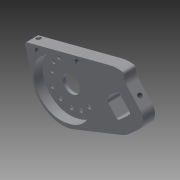
# Autodesk Inventor part: mount_alt_2015
Saved by Autodesk Inventor 2015 (Build 190159000, 159)
## iProperties
Created: 2014-05-15
Part Number: mount_alt_2015
Material: Generic
Document SubType Name: Modeling
Designer: brent
Density: 1 g/cm^3
Appearance: Default
Author: brent
Autodesk Inventor part; units mm, degrees
ref_plane "YZ Plane" through (0, 0, 0) normal (1, 0, 0) x (0, 1, 0)
ref_plane "XZ Plane" through (0, 0, 0) normal (0, 1, 0) x (-1, 0, 0)
ref_plane "XY Plane" through (0, 0, 0) normal (0, 0, 1) x (1, 0, 0)
derived "mountsketch_alt.ipt"
sketch "Sketch1" plane through (0, 0, 0) normal (0, 0, 1) x (1, 0, 0)
  circle A0 centre (-32.7716, 175.7429) radius 9 projected
  circle A1 centre (-51.4977, 187.2899) radius 2.15 projected
  circle A2 centre (-32.7716, 175.7429) radius 33 projected
  circle A3 centre (-44.3186, 157.0168) radius 2.15 projected
  circle A4 centre (-14.0455, 164.1958) radius 2.15 projected
  circle A5 centre (-21.2245, 194.4689) radius 2.15 projected
  line L0 (127, 127.3759) -> (61.9125, 127.3759) projected
  line L1 (-105.8581, 0) -> (165.8097, 0) projected
  line L2 (32.8717, 216.1784) -> (58.0256, 188.2421) projected
  line L3 (58.0256, 188.2421) -> (34.4308, 166.9972) projected
  line L4 (-21.2245, 194.4689) -> (-14.0455, 164.1958) projected
  line L5 (-32.7716, 175.7429) -> (26.1158, 189.7076) projected
  line L6 (26.1158, 189.7076) -> (-31.1651, 176.1238) projected
  circle A6 centre (-9.2209, 174.5577) radius 2.15 projected
  line L7 (26.1158, 189.7076) -> (-34.378, 175.3619) projected
  circle A7 centre (-22.6931, 156.7216) radius 2.15 projected
  circle A8 centre (-29.599, 198.068) radius 2.15 projected
  circle A9 centre (-53.1093, 177.6899) radius 2.15 projected
  circle A10 centre (-32.7312, 154.1796) radius 2.15 projected
  circle A11 centre (-15.7377, 187.0468) radius 2.15 projected
  circle A12 centre (-46.063, 194.0022) radius 2.15 projected
  circle A13 centre (-53.0184, 163.6769) radius 2.15 projected
  line L8 (16.1602, 187.2887) -> (24.9131, 177.5677) projected
  line L9 (25.6305, 177.5301) -> (38.2774, 188.9173) projected
  line L10 (38.315, 189.6348) -> (29.5621, 199.3558) projected
  line L11 (32.8717, 216.1784) -> (-36.3872, 208.5442) projected
  line L12 (34.4308, 166.9972) -> (-20.5563, 145.0869) projected
  circle A14 centre (26.1158, 189.7076) radius 34.33 projected
  line L13 (32.8717, 216.1784) -> (32.0626, 223.5186) projected
  line L14 (26.8329, 203.9052) -> (40.0897, 189.182) projected
  line L15 (16.1602, 187.2887) -> (25.9328, 176.4351) projected
  line L16 (25.9328, 176.4351) -> (40.0897, 189.182) projected
  line L17 (26.8329, 203.9052) -> (19.3412, 197.1596) projected
  ellipse E0 centre (22.8611, 193.3223) end of major axis (29.5621, 199.3558) minor radius 5.2071 (19.3412, 197.1596) -> (16.1602, 187.2887) ccw projected
  line L18 (-41.0899, 207.6772) -> (17.4623, 222.929) projected
  line L19 (-41.0899, 207.6772) -> (-73.0243, 199.3589) projected
  line L20 (-73.0243, 199.3589) -> (-64.706, 167.4245) projected
  point P0 (0, 0)
  point P1 (-2.1526, 151.7421)
  point P2 (-5.3493, 194.1009)
  point P3 (0.5466, 212.6153)
  constraints: 4 other
extrude "Extrusion11" add sketch "Sketch1" along normal blind 12.7 contours A2 A14 | L11 A14 A2 | A2 L18 A14 L11 | A2 L20 L19 | A14 L11 L2 L3 L12 A2 | A2 L5 A14 | A14 L13 L11 | A2 A14 L5 | A2 A14 L12
fillet "Fillet7" radius 25.4 1 edges at (34.4308, 166.9972, 6.35)
fillet "Fillet7" radius 2.54 1 edges at (32.0626, 223.5186, 6.35)
fillet "Fillet7" radius 12.7 2 edges at (58.0256, 188.2421, 6.35) (32.8717, 216.1784, 6.35)
sketch "Sketch17" plane through (-32.7716, 175.7429, 12.7) normal (0, 0, 1) x (0.4514581, 0.8922923, 0)
  circle A0 centre (9.5746, -21.5491) radius 2.15 projected
  circle A1 centre (0, 0) radius 9 projected
  circle A2 centre (-12.4225, -17.5803) radius 2.15 projected
  circle A3 centre (-19.9069, 12.6188) radius 2.15 projected
  circle A4 centre (10.2922, 20.1032) radius 2.15 projected
  circle A5 centre (17.7766, -10.0959) radius 2.15 projected
  circle A6 centre (-19.2225, -9.7709) radius 2.15 projected
  circle A7 centre (-7.4443, 19.0262) radius 2.15 projected
  circle A8 centre (21.3528, 7.248) radius 2.15 projected
  circle A9 centre (21.9221, -1.8493) radius 2.15 projected
  circle A10 centre (-1.8493, -21.9221) radius 2.15 projected
  circle A11 centre (-21.9221, 1.8493) radius 2.15 projected
  circle A12 centre (1.8493, 21.9221) radius 2.15 projected
  arc A13 (-22.1213, -18.6795) -> (22.1213, 18.6795) centre (1.0652, -1.2614) ccw
  arc A14 (22.1213, 18.6795) -> (-22.1213, -18.6795) centre (-1.0652, 1.2614) ccw
  line L0 (-21.0921, -19.9712) -> (-23.2224, -17.4484)
  line L1 (23.2224, 17.4484) -> (21.0921, 19.9712)
  point P0 (65.9055, 28.4481)
  point P1 (29.8536, 27.856)
  point P2 (5.2355, 34.1004)
  point P3 (-142.019, -108.5824)
  point P4 (3.0016, 34.3692)
  dimension "d178" = 58
  dimension "d179" = 58
  constraints: 8 point on circle, 4 end point, 4 tangent, 2 centre point, 2 coincident
  measures "d178" diameter of A14
  measures "d179" diameter of A13
sketch "Sketch12" plane through (49.5277, 197.68, 12.7) normal (0.7431448, 0.6691306, 0) x (0, 0, -1)
  line L0 (12.7, 0) -> (12.7, 20.801) projected
  line L1 (12.7, 13.589) -> (12.7, 0) projected
  line L2 (12.7, 13.589) -> (0, 13.589) projected
  line L3 (0, 0) -> (0, 13.589) projected
  line L4 (12.7, 0) -> (0, 0) projected
  circle A0 centre (6.35, 9.525) radius 2.413
  line L5 (12.7, 14.605) -> (12.7, 0) projected
  line L6 (12.7, 14.605) -> (0, 14.605) projected
  line L7 (0, 0) -> (0, 14.605) projected
  line L8 (12.7, 0) -> (0, 0) projected
  point P0 (12.7, -113.7644)
  dimension "d99" = 4.826
  dimension "d122" = 6.35
  dimension "d123" = 5.08
  constraints: 1 centre point
  measures "d99" diameter of A0
  measures "d122" distance from line of L0 A0.centre
  measures "d123" distance from line of L6 A0.centre
sketch "Sketch13" plane through (48.5877, 179.7441, 0) normal (0.6691306, -0.7431448, 0) x (0.7431448, 0.6691306, 0)
  line L0 (-14.5085, 12.7) -> (0, 12.7) projected
  line L1 (-18.034, 0) -> (0, 0) projected
  line L2 (-18.034, 0) -> (-18.034, 12.7) projected
  line L3 (0, 12.7) -> (-18.034, 12.7) projected
  line L4 (0, 0) -> (0, 12.7) projected
  circle A0 centre (-9.017, 6.35) radius 2.413
  point P0 (-156.38, 0)
  dimension "d100" = 4.826
  dimension "d101" = 9.017
  dimension "d102" = 6.35
  constraints: 1 centre point
  measures "d100" diameter of A0
  measures "d101" distance from line of A0.centre L4
  measures "d102" distance from line of A0.centre L0
extrude "Extrusion13" cut sketch "Sketch13" against normal blind 25.4 contours A0
extrude "Extrusion14" cut sketch "Sketch12" against normal blind 25.4 contours A0
thread "Thread5" size "10-32 UNF" class "2B" standard "ANSI Unified Screw Threads" full length
thread "Thread6" size "10-32 UNF" class "2B" standard "ANSI Unified Screw Threads" full length
sketch "Sketch16" plane through (-32.7716, 175.7429, 0) normal (0, 0, -1) x (-0.4514581, -0.8922923, 0)
  line L0 (-38.0971, 0.9443) -> (-44.0427, -11.275) projected
  line L1 (-44.0427, -11.275) -> (-60.259, -3.3847) projected
  line L2 (-60.259, -3.3847) -> (-54.3134, 8.8346) projected
  arc A0 (-64.2386, -44.1331) -> (-64.2386, -44.1331) centre (-76.0821, -48.718) ccw projected
  line L3 (-56.729, -63.5313) -> (-64.2386, -44.1331) projected
  arc A1 (-56.729, -63.5313) -> (-40.3006, -70.7899) centre (-44.8855, -58.9464) ccw projected
  line L4 (-26.7706, -65.552) -> (-40.3006, -70.7899) projected
  arc A2 (-26.7706, -65.552) -> (-19.1307, -60.9069) centre (-35.9404, -41.865) ccw projected
  line L5 (21.8394, -24.7394) -> (-19.1307, -60.9069) projected
  arc A3 (21.8394, -24.7394) -> (21.8394, 24.7394) centre (0, 0) ccw projected
  line L6 (-34.7521, 29.5687) -> (-5.2355, 34.1004) projected
  circle A4 centre (-1.8493, 21.9221) radius 2.15 projected
  circle A5 centre (21.9221, 1.8493) radius 2.15 projected
  circle A6 centre (1.8493, -21.9221) radius 2.15 projected
  circle A7 centre (-21.9221, -1.8493) radius 2.15 projected
  circle A8 centre (-21.3528, 7.248) radius 2.15 projected
  circle A9 centre (7.4443, 19.0262) radius 2.15 projected
  circle A10 centre (19.2225, -9.7709) radius 2.15 projected
  circle A11 centre (-17.7766, -10.0959) radius 2.15 projected
  circle A12 centre (-10.2922, 20.1032) radius 2.15 projected
  circle A13 centre (19.9069, 12.6188) radius 2.15 projected
  circle A14 centre (12.4225, -17.5803) radius 2.15 projected
  circle A15 centre (-9.5746, -21.5491) radius 2.15 projected
  circle A16 centre (0, 0) radius 9 projected
  line L7 (-70.2544, 22.6003) -> (-60.2386, -42.6353)
  line L8 (-60.2386, -42.6353) -> (37.6257, -27.6099)
  line L9 (37.6257, -27.6099) -> (27.6099, 37.6257)
  line L10 (27.6099, 37.6257) -> (-70.2544, 22.6003)
  point P0 (-51.5181, 22.1934)
  point P1 (-5.2355, 34.1004)
  point P2 (142.019, -108.5824)
  point P3 (-29.8536, 27.856)
  point P4 (-65.9055, 28.4481)
  point P5 (-30.9895, -27.5591)
  point P6 (-69.1415, -38.0823)
  point P7 (-3.0016, 34.3692)
  dimension "d117" = 99.011
  dimension "d118" = 66
  constraints: 8 end point, 2 parallel, 1 perpendicular, 1 tangent, 9 other
  measures "d117" distance between parallel lines of L9 L7
  measures "d118" distance between parallel lines of L10 L8
extrude "Extrusion15" cut sketch "Sketch17" against normal blind 9.525 contours A14 A13
fillet "Fillet8" radius 2.3813 3 edges at (26.8329, 203.9052, 6.35) (40.0897, 189.182, 6.35) (25.9328, 176.4351, 6.35)
fillet "Fillet9" radius 2.54 1 edges at (-73.0243, 199.3589, 6.35)
sketch "Sketch18" plane through (-32.7716, 175.7429, 0) normal (0, 0, -1) x (-0.4514581, -0.8922923, 0)
  arc A0 (-56.729, -63.5313) -> (-40.3006, -70.7899) centre (-44.8855, -58.9464) ccw projected
  line L0 (-26.7706, -65.552) -> (-40.3006, -70.7899) projected
  arc A1 (-26.7706, -65.552) -> (-19.1307, -60.9069) centre (-35.9404, -41.865) ccw projected
  line L1 (21.8394, -24.7394) -> (-19.1307, -60.9069) projected
  arc A2 (21.8394, -24.7394) -> (21.8394, 24.7394) centre (0, 0) ccw projected
  line L2 (-34.7521, 29.5687) -> (-5.2355, 34.1004) projected
  arc A3 (-41.8032, 30.5011) -> (-34.7521, 29.5687) centre (-36.6794, 42.1216) ccw projected
  arc A4 (-64.7823, -23.5207) -> (-71.2503, -34.3482) centre (-39.0458, -46.2403) ccw projected
  arc A5 (-71.2503, -34.3482) -> (-70.2556, -37.3552) centre (-68.8675, -35.2281) ccw projected
  line L3 (-69.1415, -38.0823) -> (-70.2556, -37.3552) projected
  arc A6 (-64.2386, -44.1331) -> (-64.2386, -44.1331) centre (-76.0821, -48.718) ccw projected
  line L4 (-56.729, -63.5313) -> (-64.2386, -44.1331) projected
  circle A7 centre (-1.8493, 21.9221) radius 2.15 projected
  circle A8 centre (21.9221, 1.8493) radius 2.15 projected
  circle A9 centre (1.8493, -21.9221) radius 2.15 projected
  circle A10 centre (-21.9221, -1.8493) radius 2.15 projected
  circle A11 centre (-21.3528, 7.248) radius 2.15 projected
  circle A12 centre (7.4443, 19.0262) radius 2.15 projected
  circle A13 centre (19.2225, -9.7709) radius 2.15 projected
  circle A14 centre (-17.7766, -10.0959) radius 2.15 projected
  circle A15 centre (-10.2922, 20.1032) radius 2.15 projected
  circle A16 centre (19.9069, 12.6188) radius 2.15 projected
  circle A17 centre (12.4225, -17.5803) radius 2.15 projected
  circle A18 centre (0, 0) radius 9 projected
  circle A19 centre (-9.5746, -21.5491) radius 2.15 projected
  ellipse E0 centre (-40.8018, -41.7042) end of major axis (-49.2107, -44.9595) minor radius 5.2071 (-32.3929, -38.4489) -> (-42.6367, -36.831) ccw projected
  line L5 (-32.3929, -38.4489) -> (-27.98, -49.8483) projected
  arc A20 (-29.3409, -52.9286) -> (-27.98, -49.8483) centre (-30.2006, -50.708) ccw projected
  line L6 (-29.3409, -52.9286) -> (-42.6649, -58.0867) projected
  arc A21 (-45.7452, -56.7257) -> (-42.6649, -58.0867) centre (-43.5245, -55.866) ccw projected
  line L7 (-45.7452, -56.7257) -> (-51.1783, -42.6912) projected
  arc A22 (-49.8174, -39.6108) -> (-51.1783, -42.6912) centre (-48.9577, -41.8315) ccw projected
  line L8 (-49.8174, -39.6108) -> (-42.6367, -36.831) projected
  line L9 (-85.8325, -31.7522) -> (-42.1537, -81.2311)
  line L10 (-42.1537, -81.2311) -> (46.5789, -2.9)
  line L11 (46.5789, -2.9) -> (2.9, 46.5789)
  line L12 (2.9, 46.5789) -> (-85.8325, -31.7522)
  point P0 (142.019, -108.5824)
  point P1 (-65.4837, -33.2012)
  point P2 (-3.0016, 34.3692)
  dimension "d125" = 66
  dimension "d126" = 118.3605
  constraints: 8 end point, 2 parallel, 1 collinear, 1 perpendicular, 1 tangent, 8 other
  measures "d125" distance between parallel lines of L10 L12
  measures "d126" distance between parallel lines of L11 L9
sketch "Sketch19" plane through (-32.7716, 175.7429, 0) normal (0, 0, -1) x (-0.8922923, 0.4514581, 0)
  arc A0 (44.8979, 0.9958) -> (44.6747, 4.581) centre (42.9937, 2.6768) ccw projected
  line L0 (-23.5207, 64.7823) -> (44.6747, 4.581) projected
  arc A1 (-23.5207, 64.7823) -> (-34.3482, 71.2503) centre (-46.2403, 39.0458) ccw projected
  arc A2 (-34.3482, 71.2503) -> (-37.3552, 70.2556) centre (-35.2281, 68.8675) ccw projected
  arc A3 (-44.1331, 64.2386) -> (-44.1331, 64.2386) centre (-48.718, 76.0821) ccw projected
  line L1 (-63.5313, 56.729) -> (-44.1331, 64.2386) projected
  arc A4 (-63.5313, 56.729) -> (-70.7899, 40.3006) centre (-58.9464, 44.8855) ccw projected
  line L2 (-65.552, 26.7706) -> (-70.7899, 40.3006) projected
  arc A5 (-65.552, 26.7706) -> (-60.9069, 19.1307) centre (-41.865, 35.9404) ccw projected
  line L3 (-24.7394, -21.8394) -> (-60.9069, 19.1307) projected
  arc A6 (-24.7394, -21.8394) -> (24.7394, -21.8394) centre (0, 0) ccw projected
  line L4 (44.8979, 0.9958) -> (24.7394, -21.8394) projected
  ellipse E0 centre (-41.7042, 40.8018) end of major axis (-44.9595, 49.2107) minor radius 5.2071 (-38.4489, 32.3929) -> (-36.831, 42.6367) ccw projected
  line L5 (-38.4489, 32.3929) -> (-49.8483, 27.98) projected
  arc A7 (-52.9286, 29.3409) -> (-49.8483, 27.98) centre (-50.708, 30.2006) ccw projected
  line L6 (-52.9286, 29.3409) -> (-58.0867, 42.6649) projected
  arc A8 (-56.7257, 45.7452) -> (-58.0867, 42.6649) centre (-55.866, 43.5245) ccw projected
  line L7 (-56.7257, 45.7452) -> (-42.6912, 51.1783) projected
  arc A9 (-39.6108, 49.8174) -> (-42.6912, 51.1783) centre (-41.8315, 48.9577) ccw projected
  line L8 (-39.6108, 49.8174) -> (-36.831, 42.6367) projected
  circle A10 centre (0, 0) radius 9 projected
  circle A11 centre (-21.5491, 9.5746) radius 2.15 projected
  circle A12 centre (-17.5803, -12.4225) radius 2.15 projected
  circle A13 centre (12.6188, -19.9069) radius 2.15 projected
  circle A14 centre (20.1032, 10.2922) radius 2.15 projected
  circle A15 centre (-10.0959, 17.7766) radius 2.15 projected
  circle A16 centre (-9.7709, -19.2225) radius 2.15 projected
  circle A17 centre (19.0262, -7.4443) radius 2.15 projected
  circle A18 centre (7.248, 21.3528) radius 2.15 projected
  circle A19 centre (-1.8493, 21.9221) radius 2.15 projected
  circle A20 centre (-21.9221, -1.8493) radius 2.15 projected
  circle A21 centre (1.8493, -21.9221) radius 2.15 projected
  circle A22 centre (21.9221, 1.8493) radius 2.15 projected
  line L9 (-86.7588, 32.5699) -> (-43.08, 82.0488)
  line L10 (-43.08, 82.0488) -> (46.5789, 2.9)
  line L11 (46.5789, 2.9) -> (2.9, -46.5789)
  line L12 (2.9, -46.5789) -> (-86.7588, 32.5699)
  point P0 (-33.2012, 65.4837)
  point P1 (-108.5824, -142.019)
  dimension "d128" = 66
  dimension "d129" = 119.5962
  constraints: 8 end point, 3 tangent, 2 parallel, 1 collinear, 1 perpendicular, 1 point on line, 3 other
  measures "d128" distance between parallel lines of L12 L10
  measures "d129" distance between parallel lines of L11 L9
sketch "Sketch21" plane through (17.4623, 222.929, 12.7) normal (-0.2520703, 0.9677089, 0) x (0.9677089, 0.2520703, 0)
  line L0 (0, 12.7) -> (-90.966, 12.7) projected
  circle A0 centre (-87.156, 8.89) radius 2.413
  line L1 (-93.506, 12.7) -> (-93.506, 0) projected
  point P0 (-73.0922, 12.7)
  dimension "d138" = 4.826
  dimension "d140" = 3.81
  dimension "d167" = 6.35
  constraints: 1 centre point
  measures "d138" diameter of A0
  measures "d140" distance from line of A0.centre L0
  measures "d167" distance from line of L1 A0.centre
extrude "Extrusion17" cut sketch "Sketch21" against normal blind 12.7
thread "Thread7" size "10-32 UNF" class "2B" standard "ANSI Unified Screw Threads" full length
sketch "Sketch22" plane through (-32.7716, 175.7429, 0) normal (0, 0, -1) x (-0.8922923, 0.4514581, 0)
  arc A0 (-23.5207, 64.7823) -> (-34.3482, 71.2503) centre (-46.2403, 39.0458) ccw projected
  circle A1 centre (0, 0) radius 9 projected
  circle A2 centre (-46.2403, 39.0458) radius 31.83
  circle A3 centre (0, 0) radius 11.935
  line L0 (10.2698, 6.0808) -> (-18.8514, 55.263)
  line L1 (-57.6401, 9.3272) -> (-4.2745, -11.1433)
  circle A4 centre (0, 0) radius 28
  circle A5 centre (1.1541, 36.6473) radius 2.413
  circle A6 centre (33.9061, 7.7345) radius 2.413
  line L2 (0, 0) -> (-46.2403, 39.0458)
  line L3 (-23.5207, 64.7823) -> (44.6747, 4.581) projected
  line L4 (44.8979, 0.9958) -> (24.7394, -21.8394) projected
  point P0 (-108.5824, -142.019)
  dimension "d146" = 63.66
  dimension "d147" = 23.87
  dimension "d148" = 56
  dimension "d149" = 4.826
  dimension "d150" = 4.826
  dimension "d181" = 12.7
  dimension "d182" = 4.7625
  dimension "d184" = 4.7625
  dimension "d185" = 43.688
  constraints: 6 end point, 5 centre point, 4 point on circle, 4 tangent, 3 coincident
  measures "d146" diameter of A2
  measures "d147" diameter of A3
  measures "d148" diameter of A4
  measures "d149" diameter of A5
  measures "d150" diameter of A6
  measures "d181" distance from line of L4 A6.centre
  measures "d182" distance from line of L3 A6.centre
  measures "d184" distance from line of L3 A5.centre
  measures "d185" distance of A6.centre A5.centre
extrude "Extrusion18" cut sketch "Sketch22" against normal through all contours A5 | A6
chamfer "Chamfer1" distance 2.2 angle 45 12 edges at (-31.749, 198.068, 0) (-48.213, 194.0022, 0) (-53.6477, 187.2899, 0) (-55.2593, 177.6899, 0) (-55.1684, 163.6769, 0) (-46.4686, 157.0168, 0) (-34.8812, 154.1796, 0) (-24.8431, 156.7216, 0) (-16.1955, 164.1958, 0) (-11.3709, 174.5577, 0) (-17.8877, 187.0468, 0) (-23.3745, 194.4689, 0)
thread "Thread12" size "10-32 UNF" class "2B" standard "ANSI Unified Screw Threads" full length
thread "Thread13" size "10-32 UNF" class "2B" standard "ANSI Unified Screw Threads" full length
sketch "Sketch26" plane through (-64.706, 167.4245, 0) normal (-0.9677089, -0.2520703, 0) x (0, 0, 1)
  line L0 (12.7, 30.46) -> (12.7, 0) projected
  line L1 (1.397, 33) -> (6.223, 33) projected
  line L2 (12.7, 30.6505) -> (12.7, 25.8245) projected
  line L3 (0, 25.8245) -> (12.7, 25.8245) projected
  line L4 (0, 30.6505) -> (12.7, 30.6505) projected
  circle A0 centre (8.89, 22.0145) radius 2.413
  point P0 (0, -178.3287)
  dimension "d192" = 4.826
  dimension "d193" = 3.81
  dimension "d194" = 3.81
  constraints: 1 centre point
  measures "d192" diameter of A0
  measures "d193" distance from line of L0 A0.centre
  measures "d194" distance from line of A0.centre L3
extrude "Extrusion21" cut sketch "Sketch26" against normal blind 25.4
thread "Thread14" size "10-32 UNF" class "2B" standard "ANSI Unified Screw Threads" full length
equation "\"d91\" = mount_thickness"
equation "\"d120\" = mount_thickness - mount_motor_thickness"
equation "\"mount_thickness\" = 12.7"
equation "\"mount_motor_thickness\" = 3.175"
body "Solid1"
body "Solid3"
